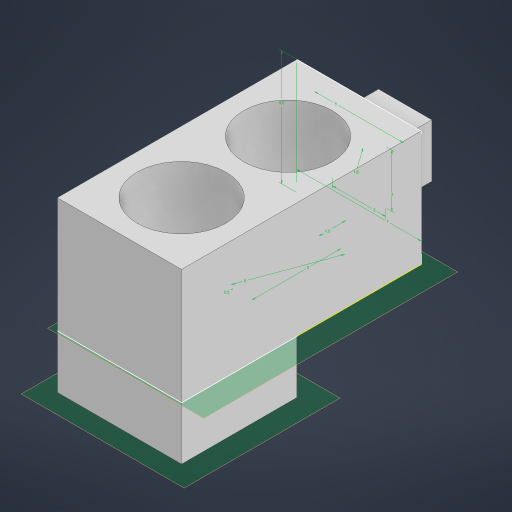
# Autodesk Inventor part: sensorholder_2
Saved by Autodesk Inventor 2023.4 (Build 274418000, 418)
## iProperties
Created: 2024-12-09
Part Number: sensorholder_2
Material: 一般
Document SubType Name: Modeling
Designer: IshiiLabHonda
Density: 1 g/cm^3
Appearance: 既定
Author: IshiiLabHonda
Autodesk Inventor part; units mm, degrees
ref_plane "YZ Plane" through (0, 0, 0) normal (1, 0, 0) x (0, 1, 0)
ref_plane "XZ Plane" through (0, 0, 0) normal (0, 1, 0) x (-1, 0, 0)
ref_plane "XY Plane" through (0, 0, 0) normal (0, 0, 1) x (1, 0, 0)
sketch "スケッチ1" plane through (0, 0, 0) normal (0, 0, 1) x (1, 0, 0)
  line L0 (-3.5, 3.25) -> (3.5, 3.25)
  line L1 (3.5, 3.25) -> (3.5, -3.25)
  line L2 (3.5, -3.25) -> (-3.5, -3.25)
  line L3 (-3.5, -3.25) -> (-3.5, 3.25)
  line L4 (-3.5, 3.25) -> (3.5, -3.25) construction
  line L5 (3.5, 3.25) -> (-3.5, -3.25) construction
  line L6 (-2.5, 3.25) -> (-2.5, -3.25) construction
  line L7 (2.5, 3.25) -> (2.5, -3.25) construction
  line L8 (0, 0) -> (0, 0.4773) construction
  line L9 (0, 0) -> (0.5273, 0) construction
  line L10 (-1.5, 1.5) -> (1.5, 1.5)
  line L11 (1.5, 1.5) -> (1.5, -1.5)
  line L12 (1.5, -1.5) -> (-1.5, -1.5)
  line L13 (-1.5, -1.5) -> (-1.5, 1.5)
  line L14 (-1.5, 1.5) -> (1.5, -1.5) construction
  line L15 (1.5, 1.5) -> (-1.5, -1.5) construction
  circle A0 centre (0, 0) radius 0.8
  dimension "d0" = 7
  dimension "d1" = 6.5
  dimension "d2" = 5
  dimension "d22" = 3
  dimension "d23" = 3
  dimension "d24" = 1.6
  constraints: 32 end point, 5 parallel, 5 perpendicular, 4 midpoint, 4 point on line, 1 centre point, 1 coincident, 1 vertical, 1 other
  measures "d0" distance of L0.start L0.end
  measures "d1" distance of L2.end L0.start
  measures "d2" distance between parallel lines of L6 L7
  measures "d22" distance of L11.end L12.end
  measures "d23" distance of L10.end L11.end
  measures "d24" diameter of A0
extrude "押し出し1" add sketch "スケッチ1" along normal blind 13.5 contours L0 L1 L2 L3 | L10 L11 L12 L13 | A0
ref_plane "作業平面1" through (-3.5, -3.25, 0) normal (0, -1, 0) x (1, 0, 0)
sketch "スケッチ2" plane through (-3.5, -3.25, 0) normal (0, -1, 0) x (1, 0, 0)
  line L0 (0, 0) -> (7, 0) projected
  line L1 (7, 0) -> (7, 13.5) projected
  line L2 (0, 13.5) -> (7, 13.5) projected
  line L3 (0, 0) -> (0, 13.5) projected
  line L4 (0, 0) -> (0, 13.5) projected
  line L5 (7, 0) -> (7, 13.5) projected
  line L6 (0, 0) -> (7, 0) projected
  line L7 (0, 0) -> (0, 13.5) projected
  line L8 (0, 1.5) -> (7, 1.5) construction
  line L9 (0, 6.5) -> (7, 6.5) construction
  line L10 (7, 0) -> (7, 13.5) projected
  line L11 (0, 6.5) -> (7, 1.5) construction
  line L12 (7, 6.5) -> (0, 1.5) construction
  circle A0 centre (3.5, 4) radius 2.5
  line L13 (0, 7) -> (7, 7)
  line L14 (0, 7) -> (0, 13.5)
  line L15 (0, 13.5) -> (7, 13.5) projected
  line L16 (7, 13.5) -> (7, 7)
  line L17 (7, 13.5) -> (0, 13.5)
  point P0 (3.5, 0)
  point P1 (0, 7)
  point P2 (7, 7)
  dimension "d8" = 1.5
  dimension "d9" = 5
  dimension "d10" = 5
  dimension "d11" = 0.5
  constraints: 16 end point, 6 point on line, 4 perpendicular, 2 collinear, 1 centre point, 1 midpoint
  measures "d8" distance between parallel lines of L0 L8
  measures "d9" distance between parallel lines of L8 L9
  measures "d10" diameter of A0
  measures "d11" distance between parallel lines of L9 L13
extrude "押し出し2" add sketch "スケッチ2" along normal blind 3 contours L3 L2 L1 L13
ref_plane "作業平面2" through (-3.5, -6.25, 0) normal (0, -1, 0) x (1, 0, 0)
sketch "スケッチ3" plane through (-3.5, -6.25, 0) normal (0, -1, 0) x (1, 0, 0)
  line L0 (7, 7) -> (7, 13.5) projected
  line L1 (7, 13.5) -> (0, 13.5) projected
  line L2 (0, 13.5) -> (0, 7) projected
  line L3 (0, 7) -> (7, 7) projected
  line L4 (0, 0) -> (0, 13.5) projected
  line L5 (7, 7) -> (7, 13.5) projected
  line L6 (0, 7) -> (7, 7) projected
  line L7 (0, 7.5) -> (7, 7.5) construction
  line L8 (7, 0) -> (7, 13.5) projected
  line L9 (0, 12.5) -> (7, 12.5) construction
  line L10 (0, 12.5) -> (7, 7.5) construction
  line L11 (7, 12.5) -> (0, 7.5) construction
  circle A0 centre (3.5, 10) radius 2.5
  point P0 (3.5, 0)
  dimension "d15" = 0.5
  dimension "d16" = 1
  dimension "d17" = 5
  constraints: 8 end point, 4 point on line, 1 centre point, 1 midpoint, 1 parallel, 1 perpendicular
  measures "d15" distance between parallel lines of L3 L7
  measures "d16" distance between parallel lines of L1 L9
  measures "d17" diameter of A0
extrude "押し出し3" cut sketch "スケッチ3" against normal up to surface (9.5 mm away) contours A0
extrude "押し出し4" cut sketch "スケッチ2" against normal blind 10 contours A0
extrude "押し出し5" add sketch "スケッチ1" against normal blind 2.6 contours L10 L11 L12 L13 | A0
